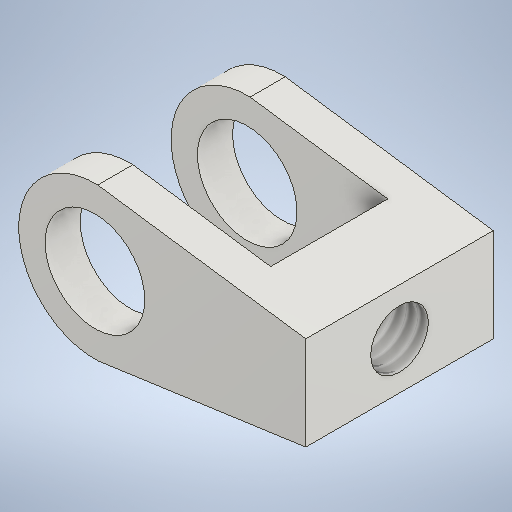
# Autodesk Inventor part: 16C - Con Head Crosshead
Saved by Autodesk Inventor 2025.2 (Build 292293000, 293)
## iProperties
Created: 2025-06-12
Part Number: 16C - Con Head Crosshead
Material: Steel AISI 1020 107 HR
Document SubType Name: Modeling
Designer: bless
Density: 7.87 g/cm^3
Appearance: Steel
Author: bless
Autodesk Inventor part; units mm, degrees
ref_plane "YZ Plane" through (0, 0, 0) normal (1, 0, 0) x (0, 1, 0)
ref_plane "XY Plane" through (0, 0, 0) normal (0, 0, 1) x (1, 0, 0)
sketch "Sketch1" plane through (0, 0, 0) normal (0, 0, 1) x (1, 0, 0)
  arc A0 (0.2442, 6.4954) -> (0.2442, -6.4954) centre (0, 0) ccw
  line L0 (18, 4) -> (18, -4)
  line L1 (18, 4) -> (0.2442, 6.4954)
  line L2 (0.2442, -6.4954) -> (18, -4)
  point P0 (18, 0)
  dimension "d0" = 13
  dimension "d1" = 8
  dimension "d2" = 18
  dimension "d3" = 82
  dimension "d4" = 82
  constraints: 6 end point, 2 point on circle, 1 centre point, 1 coincident, 1 horizontal alignment, 1 midpoint, 1 vertical
  measures "d0" diameter of A0
  measures "d1" distance of L0.start L0.end
  measures "d2" distance from line of L0 point (0, 0)
  measures "d3" angle of L0 L2
  measures "d4" angle of L0 L1
extrude "Extrusion1" add sketch "Sketch1" along normal blind 16
sketch "Sketch2" plane through (0, 0, 16) normal (0, 0, 1) x (1, 0, 0)
  arc A0 (0.2442, 6.4954) -> (0.2442, -6.4954) centre (0, 0) ccw projected
  circle A1 centre (0, 0) radius 4.25
  dimension "d7" = 8.5
  constraints: 1 centre point, 1 coincident
  measures "d7" diameter of A1
extrude "Extrusion2" cut sketch "Sketch2" against normal through all
ref_plane "Work Plane1" through (0, 6.5, 0) normal (0, 1, 0) x (-1, 0, 0)
sketch "Sketch3" plane through (0, 6.5, 0) normal (0, 1, 0) x (-1, 0, 0)
  line L0 (6.5, 0) -> (6.5, 16) projected
  line L1 (6.5, 13) -> (-12, 13)
  line L2 (-12, 13) -> (-12, 3)
  line L3 (-12, 3) -> (6.5, 3)
  line L4 (6.5, 3) -> (6.5, 13)
  line L5 (-18, 0) -> (-18, 16) projected
  line L6 (6.5, 0) -> (-0.2442, 0) projected
  line L7 (6.5, 16) -> (-0.2442, 16) projected
  point P0 (0, 0)
  point P1 (6.5, 3)
  dimension "d11" = 6
  dimension "d12" = 3
  dimension "d13" = 3
  constraints: 8 end point, 2 parallel, 1 horizontal, 1 perpendicular, 1 point on line
  measures "d11" distance between parallel lines of L2 L5
  measures "d12" distance between parallel lines of L6 L3
  measures "d13" distance between parallel lines of L7 L1
extrude "Extrusion3" cut sketch "Sketch3" against normal through all
sketch "Sketch4" plane through (12, -4.8432, 3) normal (-1, 0, 0) x (0, 0, 1)
  line L0 (10, 9.6865) -> (10, 0) projected
  circle A0 centre (5, 4.8432) radius 2.5
  line L1 (-3, 8.8432) -> (13, 8.8432) projected
  point P0 (-3, 4.8432)
  dimension "d16" = 5
  dimension "d17" = 4
  dimension "d18" = 5
  constraints: 1 centre point
  measures "d16" diameter of A0
  measures "d17" distance from line of L1 A0.centre
  measures "d18" distance from line of A0.centre L0
hole "Hole1" at (12, 0, 8) direction (1, 0, 0) diameter 4.917 depth 6 thread size "M6x1" class "6H" standard "ANSI Metric M Profile"
body "Solid1"
